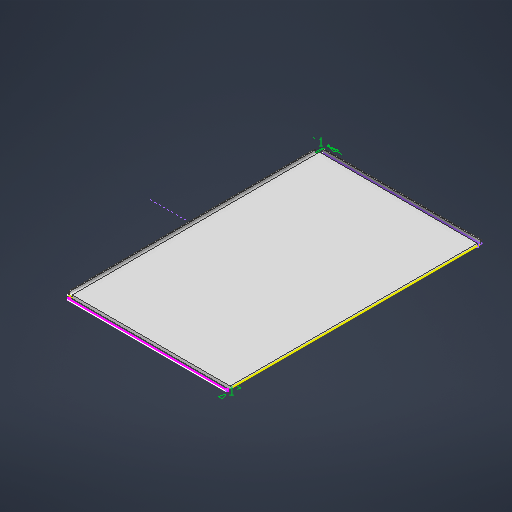
# Autodesk Inventor part: 트리보_구라뚜껑_quarter2
Saved by Autodesk Inventor 2026.2 (Build 302298010, 298A)
## iProperties
Created: 2026-06-17
Part Number: 트리보_구라뚜껑_quarter2
Material: 일반
Document SubType Name: Modeling
Designer: User
Density: 1 g/cm^3
Appearance: 기본값
Author: User
Autodesk Inventor part; units mm, degrees
ref_plane "YZ Plane" through (0, 0, 0) normal (1, 0, 0) x (0, 1, 0)
ref_plane "XZ Plane" through (0, 0, 0) normal (0, 1, 0) x (-1, 0, 0)
ref_plane "XY Plane" through (0, 0, 0) normal (0, 0, 1) x (1, 0, 0)
sketch "스케치1" plane through (0, 0, 0) normal (0, 1, 0) x (-1, 0, 0)
  line L0 (75, 117.5) -> (-75, 117.5)
  line L1 (-75, 117.5) -> (-75, -117.5)
  line L2 (-75, -117.5) -> (75, -117.5)
  line L3 (75, -117.5) -> (75, 117.5)
  line L4 (75, 117.5) -> (-75, -117.5) construction
  line L5 (-75, 117.5) -> (75, -117.5) construction
  line L6 (75, 117.5) -> (-75, 117.5)
  line L7 (-75, 117.5) -> (-75, 120.45)
  line L8 (-75, 120.45) -> (75, 120.45)
  line L9 (75, 120.45) -> (75, 117.5)
  line L10 (75, 117.5) -> (77.95, 117.5)
  line L11 (77.95, 117.5) -> (77.95, -117.5)
  line L12 (77.95, -117.5) -> (75, -117.5)
  line L13 (75, -117.5) -> (75, 117.5)
  line L14 (0, 0) -> (112, 0) construction
  line L15 (75, -117.5) -> (-75, -117.5)
  line L16 (75, -117.5) -> (-75, -117.5)
  line L17 (-75, -117.5) -> (-75, -120.45)
  line L18 (-75, -120.45) -> (75, -120.45)
  line L19 (75, -120.45) -> (75, -117.5)
  line L20 (75, -117.5) -> (77.95, -117.5)
  dimension "d0" = 235
  dimension "d1" = 150
  dimension "d7" = 2.95
  dimension "d8" = 2.95
  constraints: 42 end point, 6 parallel, 4 horizontal, 4 symmetric about line, 3 perpendicular, 2 midpoint, 1 point on line
  measures "d0" distance of L2.end L0.start
  measures "d1" distance of L0.start L0.end
  measures "d7" distance of L6.end L7.end
  measures "d8" distance of L11.end L12.end
extrude "돌출1" add sketch "스케치1" along normal blind 1 contours L10 L11 L12 L3 | L19 L18 L17 L2
extrude "돌출2" add sketch "스케치1" along normal blind 3 contours L3 L2 L1 L0
sketch "스케치3" plane through (0, 1, 0) normal (0, 1, 0) x (1, 0, 0)
  line L0 (-75, -120.45) -> (75, -120.45) projected
  line L1 (-75, -120.45) -> (75, -120.45)
  line L2 (75, -120.45) -> (75, -121.45)
  line L3 (75, -121.45) -> (-75, -121.45)
  line L4 (-75, -121.45) -> (-75, -120.45)
  line L5 (-77.95, -117.5) -> (-75, -117.5) projected
  line L6 (-77.95, -117.5) -> (-78.95, -117.5)
  line L7 (-78.95, -117.5) -> (-78.95, 117)
  line L8 (-78.95, 117) -> (-77.95, 117)
  line L9 (-77.95, 117) -> (-77.95, -117.5)
  line L10 (75, -117.5) -> (75, 120.45) projected
  line L11 (75, 0) -> (-120, 0) construction
  line L12 (-75, 120.45) -> (75, 120.45)
  line L13 (-75, 120.45) -> (75, 120.45)
  line L14 (75, 120.45) -> (75, 121.45)
  line L15 (75, 121.45) -> (-75, 121.45)
  line L16 (-75, 121.45) -> (-75, 120.45)
  line L17 (-77.95, 117.5) -> (-75, 117.5)
  line L18 (-77.95, 117.5) -> (-78.95, 117.5)
  point P0 (0, 0)
  point P1 (75, 117.5)
  dimension "d11" = 1
  dimension "d12" = 1
  constraints: 32 end point, 9 symmetric about line, 4 parallel, 3 horizontal, 2 perpendicular, 1 point on line
  measures "d11" distance of L1.end L2.end
  measures "d12" distance of L7.end L8.end
extrude "돌출3" add sketch "스케치3" along normal blind 3 contours L6 L7 L8 L9 | L16 L15 L14 L12
